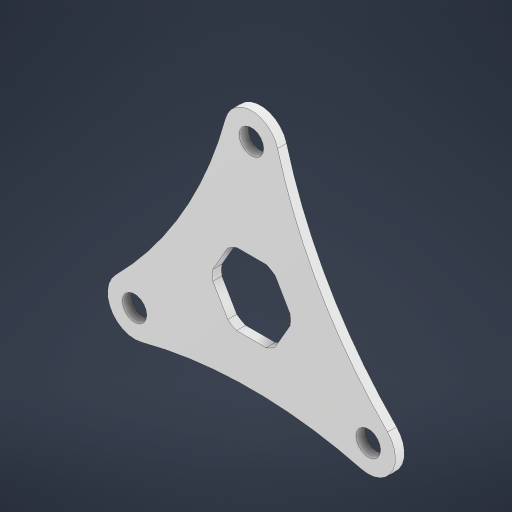
# Autodesk Inventor part: flex_wheel_hub
Saved by Autodesk Inventor 2024 (Build 280153000, 153)
## iProperties
Created: 2023-10-29
Part Number: flex_wheel_hub
Material: Acetal Resin, White
Document SubType Name: Modeling
Designer: avere
Density: 1.425 g/cm^3
Appearance: Smooth - White
Author: avere
Autodesk Inventor part; units mm, degrees
ref_plane "YZ Plane" through (0, 0, 0) normal (1, 0, 0) x (0, 1, 0)
ref_plane "XZ Plane" through (0, 0, 0) normal (0, 1, 0) x (-1, 0, 0)
ref_plane "XY Plane" through (0, 0, 0) normal (0, 0, 1) x (1, 0, 0)
sketch "VersaHex Adapter Hole" plane through (0, 0, 0) normal (0, 0, 1) x (1, 0, 0)
  line L0 (-2.6931, -2.4859) -> (-0.0712, 2.0554)
  arc A0 (1.4952, 2.9597) -> (-0.0712, 2.0554) centre (4.1171, -3.3903) ccw
  line L1 (1.4952, 2.9597) -> (6.7391, 2.9597)
  arc A1 (8.3055, 2.0554) -> (6.7391, 2.9597) centre (4.1171, -3.3903) ccw
  line L2 (8.3055, 2.0554) -> (10.9274, -2.4859)
  arc A2 (10.9274, -4.2946) -> (10.9274, -2.4859) centre (4.1171, -3.3903) ccw
  line L3 (10.9274, -4.2946) -> (8.3055, -8.8359)
  arc A3 (6.7391, -9.7403) -> (8.3055, -8.8359) centre (4.1171, -3.3903) ccw
  line L4 (6.7391, -9.7403) -> (1.4952, -9.7403)
  arc A4 (-0.0712, -8.8359) -> (1.4952, -9.7403) centre (4.1171, -3.3903) ccw
  line L5 (-0.0712, -8.8359) -> (-2.6931, -4.2946)
  arc A5 (-2.6931, -2.4859) -> (-2.6931, -4.2946) centre (4.1171, -3.3903) ccw
  point P0 (3.8427, -3.1642)
  point P1 (0, 3.175)
  point P2 (0, -3.175)
  point P3 (0, 0)
sketch "Block2" plane through (0, 0, 0) normal (0, 0, 1) x (1, 0, 0)
  line L0 (30.4112, -18.6542) -> (33.0331, -14.1129)
  arc A0 (34.5995, -13.2085) -> (33.0331, -14.1129) centre (37.2214, -19.5585) ccw
  line L1 (34.5995, -13.2085) -> (39.8433, -13.2085)
  arc A1 (41.4097, -14.1129) -> (39.8433, -13.2085) centre (37.2214, -19.5585) ccw
  line L2 (41.4097, -14.1129) -> (44.0316, -18.6542)
  arc A2 (44.0316, -20.4629) -> (44.0316, -18.6542) centre (37.2214, -19.5585) ccw
  line L3 (44.0316, -20.4629) -> (41.4097, -25.0042)
  arc A3 (39.8433, -25.9085) -> (41.4097, -25.0042) centre (37.2214, -19.5585) ccw
  line L4 (39.8433, -25.9085) -> (34.5995, -25.9085)
  arc A4 (33.0331, -25.0042) -> (34.5995, -25.9085) centre (37.2214, -19.5585) ccw
  line L5 (33.0331, -25.0042) -> (30.4112, -20.4629)
  arc A5 (30.4112, -18.6542) -> (30.4112, -20.4629) centre (37.2214, -19.5585) ccw
  point P0 (37.2214, -19.5585)
sketch "Sketch1" plane through (0, 0, 0) normal (0, 0, 1) x (1, 0, 0)
  circle A0 centre (-20.6222, -11.9063) radius 2.1526
  circle A1 centre (20.6222, -11.9062) radius 2.1526
  circle A2 centre (0, 23.8125) radius 2.1526
  arc A3 (-24.0046, -8.5535) -> (-19.4099, -16.5119) centre (-20.6222, -11.9063) ccw
  arc A4 (19.4099, -16.5119) -> (24.0046, -8.5535) centre (20.6222, -11.9062) ccw
  arc A5 (4.5947, 25.0654) -> (-4.5947, 25.0654) centre (0, 23.8125) ccw
  arc A6 (19.4099, -16.5119) -> (-19.4099, -16.5119) centre (0, -90.2489) ccw
  arc A7 (-24.0046, -8.5535) -> (-4.5947, 25.0654) centre (-78.1579, 45.1245) ccw
  arc A8 (4.5947, 25.0654) -> (24.0046, -8.5535) centre (78.1579, 45.1245) ccw
  line L0 (-6.8102, 0.9044) -> (-4.1883, 5.4456)
  arc A9 (-2.6219, 6.35) -> (-4.1883, 5.4456) centre (0, 0) ccw
  line L1 (-2.6219, 6.35) -> (2.6219, 6.35)
  arc A10 (4.1883, 5.4456) -> (2.6219, 6.35) centre (0, 0) ccw
  line L2 (4.1883, 5.4456) -> (6.8102, 0.9044)
  arc A11 (6.8102, -0.9044) -> (6.8102, 0.9044) centre (0, 0) ccw
  line L3 (6.8102, -0.9044) -> (4.1883, -5.4456)
  arc A12 (2.6219, -6.35) -> (4.1883, -5.4456) centre (0, 0) ccw
  line L4 (2.6219, -6.35) -> (-2.6219, -6.35)
  arc A13 (-4.1883, -5.4456) -> (-2.6219, -6.35) centre (0, 0) ccw
  line L5 (-4.1883, -5.4456) -> (-6.8102, -0.9044)
  arc A14 (-6.8102, 0.9044) -> (-6.8102, -0.9044) centre (0, 0) ccw
  dimension "d5" = 9.525
  dimension "d6" = 9.525
  dimension "d7" = 9.525
  constraints: 12 point on circle, 9 centre point, 6 tangent, 3 coincident, 3 other
  measures "d5" diameter of A3
  measures "d6" diameter of A4
  measures "d7" diameter of A5
extrude "Extrusion1" add sketch "Sketch1" along normal blind 1.5875
body "Solid1"
